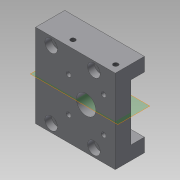
# Autodesk Inventor part: connection_hand_2
Saved by Autodesk Inventor 2017 (Build 210142000, 142)
## iProperties
Part Number: connection_hand_2
Material: Aluminium 6061
Document SubType Name: Modeling
Designer: Max
Density: 2.7 g/cm^3
Appearance: Vorgabe
Mass: 44.4667 g
Surface Area: 72.1816 cm^2
Volume: 16.4691 cm^3
Author: Max
Autodesk Inventor part; units mm, degrees
ref_plane "YZ Plane" through (0, 0, 0) normal (1, 0, 0) x (0, 1, 0)
ref_plane "XZ Plane" through (0, 0, 0) normal (0, 1, 0) x (-1, 0, 0)
ref_plane "XY Plane" through (0, 0, 0) normal (0, 0, 1) x (1, 0, 0)
sketch "Skizze1" plane through (0, 0, 0) normal (0, 1, 0) x (-1, 0, 0)
  line L0 (-34, 21.5) -> (34, 21.5)
  line L1 (34, 21.5) -> (34, -21.5)
  line L2 (34, -21.5) -> (-34, -21.5)
  line L3 (-34, -21.5) -> (-34, 21.5)
  line L4 (-34, 21.5) -> (34, -21.5) construction
  line L5 (34, 21.5) -> (-34, -21.5) construction
  point P0 (0, 0)
  dimension "d0" = 43
  dimension "d1" = 68
  constraints: 12 end point, 2 midpoint, 2 parallel, 1 horizontal, 1 perpendicular
  measures "d0" distance of L0.end L1.end
  measures "d1" distance of L1.end L2.end
extrude "Extrusion1" add sketch "Skizze1" along normal blind 15
sketch "Skizze2" plane through (0, 15, 0) normal (0, 1, 0) x (1, 0, 0)
  line L0 (-34, -21.5) -> (34, -21.5) projected
  line L1 (34, -21.5) -> (34, 21.5) projected
  line L2 (34, 21.5) -> (-34, 21.5) projected
  line L3 (-34, 21.5) -> (-34, -21.5) projected
  line L4 (-34, 14.5) -> (27, 14.5)
  line L5 (27, 14.5) -> (27, -14.5)
  line L6 (27, -14.5) -> (-34, -14.5)
  line L7 (-34, -14.5) -> (-34, 14.5)
  point P0 (0, 0)
  dimension "d4" = 29
  dimension "d5" = 14.5
  dimension "d9" = 7
  dimension "d10" = 7
  constraints: 8 end point, 2 parallel, 1 horizontal, 1 perpendicular, 1 point on line
  measures "d4" distance of L4.end L5.end
  measures "d5" distance from line of L4 point (0, 0)
  measures "d9" distance between parallel lines of L2 L4
  measures "d10" distance between parallel lines of L1 L5
extrude "Extrusion2" cut sketch "Skizze2" against normal blind 7 contours L3 L4 L5 L6
sketch "Skizze3" plane through (0, 0, 0) normal (0, -1, 0) x (1, 0, 0)
  line L0 (-34, 14.5) -> (-34, -14.5) projected
  line L1 (27, 14.5) -> (-34, 14.5) projected
  line L2 (27, -14.5) -> (27, 14.5) projected
  line L3 (-34, -14.5) -> (27, -14.5) projected
  circle A0 centre (12, 0) radius 5
  line L4 (0, 0) -> (50.6239, 0) construction
  point P0 (16, 17.3)
  dimension "d11" = 11
  dimension "d12" = 17.3
  dimension "d24" = 10
  dimension "d27" = 4
  constraints: 2 end point, 1 centre point, 1 horizontal, 1 point on line
  measures "d11" distance from line of point (16, 17.3) L2
  measures "d12" vertical distance of L4.start point (16, 17.3)
  measures "d24" diameter of A0
  measures "d27" horizontal distance of point (16, 17.3) A0.centre
hole "Bohrung1" at (16, 0, 17.3) direction (0, 1, 0) diameter 3.4 end through all counterbore diameter 6.5 counterbore depth 3.4 clearance for "Inbusschraube ISO 4762" size "M3" standard "ISO"
pattern_linear "Rechteckige Anordnung1" count 3 spacing 22 along (-1, 0, 0) of "Bohrung1"
ref_plane "Arbeitsebene1" through (-34, 0, 0) normal (0, 0, 1) x (1, 0, 0)
mirror "Spiegeln1" about plane through (-34, 0, 0) normal (0, 0, 1) of "Bohrung1", "Rechteckige Anordnung1"
extrude "Extrusion3" cut sketch "Skizze3" against normal through all contours A0
sketch "Skizze4" plane through (0, 8, 0) normal (0, 1, 0) x (1, 0, 0)
  circle A0 centre (12, 0) radius 5 projected
  line L0 (-34, -14.5) -> (-34, 14.5) projected
  line L1 (27, -14.5) -> (-34, -14.5) projected
  line L2 (27, 14.5) -> (27, -14.5) projected
  line L3 (-34, 14.5) -> (27, 14.5) projected
  line L4 (21, -9) -> (3, -9)
  line L5 (3, -9) -> (3, 9)
  line L6 (3, 9) -> (21, 9)
  line L7 (21, 9) -> (21, -9)
  line L8 (21, -9) -> (3, 9) construction
  line L9 (3, -9) -> (21, 9) construction
  point P0 (0, 0)
  dimension "d28" = 18
  dimension "d29" = 18
  constraints: 12 end point, 2 midpoint, 2 parallel, 1 horizontal, 1 perpendicular
  measures "d28" distance of L4.end L5.end
  measures "d29" distance of L5.end L6.end
hole "Bohrung2" at (3, 8, 9) at (3, 8, -9) at (21, 8, -9) at (21, 8, 9) direction (0, -1, 0) diameter 2.459 depth 8.8 tip angle 118 thread size "M3x0.5" class "6H" standard "ISO Metric profile"
sketch "Skizze5" plane through (0, 15, 0) normal (0, 1, 0) x (1, 0, 0)
  circle A0 centre (-28, 17.3) radius 1.7 projected
  circle A1 centre (-6, 17.3) radius 1.7 projected
  circle A2 centre (16, 17.3) radius 1.7 projected
  circle A3 centre (-28, -17.3) radius 1.7 projected
  circle A4 centre (-6, -17.3) radius 1.7 projected
  circle A5 centre (16, -17.3) radius 1.7 projected
  line L0 (27, -14.5) -> (-34, -14.5) projected
  line L1 (-34, -14.5) -> (-34, -21.5) projected
  line L2 (-34, -21.5) -> (34, -21.5) projected
  line L3 (34, -21.5) -> (34, 21.5) projected
  line L4 (34, 21.5) -> (-34, 21.5) projected
  line L5 (-34, 21.5) -> (-34, 14.5) projected
  line L6 (-34, 14.5) -> (27, 14.5) projected
  line L7 (27, 14.5) -> (27, -14.5) projected
  line L8 (-34, 21.5) -> (34, 21.5) projected
  line L9 (34, -21.5) -> (27, -21.5)
  line L10 (27, -21.5) -> (27, 21.5)
  line L11 (27, 21.5) -> (34, 21.5)
  line L12 (34, 21.5) -> (34, -21.5)
  point P0 (0, 0)
  constraints: 8 end point, 2 parallel, 1 horizontal, 1 perpendicular, 1 point on line
extrude "Extrusion4" cut sketch "Skizze5" against normal through all contours L7 L10 L4 L3 L2
sketch "Skizze6" plane through (-34, 0, -21.5) normal (-1, 0, 0) x (0, 0, 1)
  line L0 (36, 15) -> (36, 8) projected
  line L1 (36, 8) -> (7, 8) projected
  line L2 (7, 8) -> (7, 15) projected
  line L3 (0, 15) -> (7, 15) projected
  line L4 (0, 0) -> (0, 15) projected
  line L5 (43, 0) -> (0, 0) projected
  line L6 (43, 0) -> (43, 15) projected
  line L7 (36, 15) -> (43, 15) projected
  point P0 (21.5, 0)
extrude "Extrusion5" cut sketch "Skizze6" against normal blind 20
sketch "Skizze7" plane through (27, 0, -21.5) normal (0, 0, -1) x (-1, 0, 0)
  line L0 (34.7, 3.4) -> (31.3, 3.4) projected
  line L1 (36.25, 3.4) -> (29.75, 3.4) projected
  line L2 (31.3, 15) -> (34.7, 15) projected
  line L3 (9.3, 15) -> (12.7, 15) projected
  line L4 (14.25, 3.4) -> (7.75, 3.4) projected
  line L5 (34.7, 15) -> (34.7, 3.4)
  line L6 (34.7, 3.4) -> (34.7, 15) projected
  line L7 (31.3, 15) -> (31.3, 3.4)
  line L8 (9.3, 3.4) -> (12.7, 3.4) projected
  line L9 (12.7, 15) -> (12.7, 3.4)
  line L10 (9.3, 15) -> (9.3, 3.4)
  line L11 (0, 8) -> (41, 8) projected
  line L12 (29.75, 3.4) -> (29.75, 0)
  line L13 (29.75, 0) -> (29.75, 3.4) projected
  line L14 (29.75, 3.4) -> (36.25, 3.4) projected
  line L15 (36.25, 3.4) -> (36.25, 0)
  line L16 (36.25, 0) -> (36.25, 3.4) projected
  line L17 (14.25, 3.4) -> (14.25, 0)
  line L18 (14.25, 3.4) -> (14.25, 0) projected
  line L19 (7.75, 3.4) -> (14.25, 3.4) projected
  line L20 (7.75, 3.4) -> (7.75, 0)
  line L21 (7.75, 3.4) -> (7.75, 0) projected
  line L22 (41, 0) -> (0, 0) projected
  point P0 (27, 0)
  point P1 (25.75, 4)
  point P2 (3.75, 4)
  dimension "d41" = 8
  dimension "d42" = 4
  dimension "d43" = 4
  dimension "d44" = 4
  dimension "d45" = 4
  constraints: 16 end point, 4 point on line, 2 equal length, 2 vertical
  measures "d41" distance between parallel lines of L22 L11
  measures "d42" distance from line of L11 point (25.75, 4)
  measures "d43" distance from line of L11 point (3.75, 4)
  measures "d44" distance from line of point (25.75, 4) L13
  measures "d45" distance from line of point (3.75, 4) L20
hole "Bohrung3" at (1.25, 4, -21.5) at (23.25, 4, -21.5) direction (0, 0, 1) diameter 2.459 depth 8.8 tip angle 118 thread size "M3x0.5" class "6H" standard "ISO Metric profile"
ref_plane "Arbeitsebene2" through (27, 0, 0) normal (0, 0, -1) x (-1, 0, 0)
mirror "Spiegeln2" about plane through (27, 0, 0) normal (0, 0, -1) of "Bohrung3"
equation "\"d5\" = 0.5 * d4"
equation "\"d10\" = d9"
equation "\"d29\" = d28"
equation "\"d42\" = 0.5 * d41"
equation "\"d43\" = d42"
